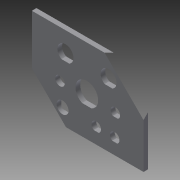
# Autodesk Inventor part: Yagi_Front_BackPlate
Saved by Autodesk Inventor 2014 (Build 180170000, 170)
## iProperties
Created: 2015-01-07
Part Number: Yagi_Front_BackPlate
Material: Generic
Document SubType Name: Modeling
Designer: Owner
Density: 1 g/cm^3
Appearance: Default
Author: Owner
Autodesk Inventor part; units mm, degrees
ref_plane "YZ Plane" through (0, 0, 0) normal (1, 0, 0) x (0, 1, 0)
ref_plane "XZ Plane" through (0, 0, 0) normal (0, 1, 0) x (-1, 0, 0)
ref_plane "XY Plane" through (0, 0, 0) normal (0, 0, 1) x (1, 0, 0)
sketch "Sketch1" plane through (0, 0, 0) normal (0, 0, 1) x (1, 0, 0)
  line L0 (-24.8346, -36.7982) -> (51.3654, -36.7982)
  line L1 (51.3654, -36.7982) -> (51.3654, -93.9482)
  line L2 (51.3654, -93.9482) -> (-24.8346, -93.9482)
  line L3 (-24.8346, -93.9482) -> (-24.8346, -36.7982)
  point P0 (0, 0)
  dimension "d0" = 76.2
  dimension "d1" = 57.15
  constraints: 8 end point, 2 parallel, 1 horizontal, 1 perpendicular
  measures "d0" distance of L0.start L0.end
  measures "d1" distance of L0.end L1.end
extrude "Extrusion1" add sketch "Sketch1" along normal blind 3.175
sketch "Sketch2" plane through (0, 0, 0) normal (0, 0, -1) x (-1, 0, 0)
  line L0 (24.8346, -93.9482) -> (24.8346, -36.7982) projected
  line L1 (-51.3654, -93.9482) -> (24.8346, -93.9482) projected
  circle A0 centre (-27.529, -50.54) radius 9.0932 construction
  arc A1 (-24.7899, -55.2644) -> (-30.2681, -55.2644) centre (-27.529, -50.54) ccw
  line L2 (-30.2681, -55.2644) -> (-24.7899, -55.2644)
  circle A2 centre (-12.6895, -67.132) radius 10.3124 construction
  arc A3 (-9.447, -74.1678) -> (-15.9319, -74.1678) centre (-12.6895, -67.132) ccw
  line L3 (-15.9319, -74.1678) -> (-9.447, -74.1678)
  circle A4 centre (1.9171, -50.54) radius 9.0932 construction
  arc A5 (4.6562, -55.2644) -> (-0.822, -55.2644) centre (1.9171, -50.54) ccw
  line L4 (-0.822, -55.2644) -> (4.6562, -55.2644)
  circle A6 centre (3.8538, -83.4188) radius 4.1
  circle A7 centre (3.8538, -83.4188) radius 5.25 construction
  line L5 (24.8346, -54.8925) -> (24.8346, -40.8771)
  line L6 (24.8346, -36.7982) -> (-51.3654, -36.7982) projected
  arc A8 (-29.9902, -86.1688) -> (-33.4543, -86.1688) centre (-31.7222, -83.4188) ccw
  line L7 (-29.9902, -86.1688) -> (-33.4543, -86.1688)
  circle A9 centre (-31.7222, -83.4188) radius 5.5 construction
  arc A10 (-30.4636, -71.2982) -> (-33.9278, -71.2982) centre (-32.1957, -68.5482) ccw
  line L8 (-30.4636, -71.2982) -> (-33.9278, -71.2982)
  circle A11 centre (-32.1957, -68.5482) radius 5.5 construction
  arc A12 (3.8538, -65.7982) -> (7.3179, -65.7982) centre (5.5858, -68.5482) ccw
  line L9 (3.8538, -65.7982) -> (7.3179, -65.7982)
  circle A13 centre (5.5858, -68.5482) radius 5.5 construction
  arc A14 (-17.3964, -86.1688) -> (-20.8605, -86.1688) centre (-19.1284, -83.4188) ccw
  line L10 (-17.3964, -86.1688) -> (-20.8605, -86.1688)
  circle A15 centre (-19.1284, -83.4188) radius 5.5 construction
  line L11 (-51.3654, -36.7982) -> (-51.3654, -93.9482) projected
  line L12 (-45.0154, -36.7982) -> (-45.0154, -93.9482) construction
  line L13 (12.1346, -93.9482) -> (12.1346, -36.7982) construction
  line L14 (-51.3654, -90.7732) -> (24.8346, -90.7732) construction
  line L15 (-51.3654, -39.9732) -> (24.8346, -39.9732) construction
  point P0 (0, 0)
  dimension "d28" = 18.1864
  dimension "d29" = 10.922
  dimension "d30" = 4.7244
  dimension "d31" = 20.6248
  dimension "d32" = 15.494
  dimension "d33" = 7.0358
  dimension "d34" = 18.1864
  dimension "d35" = 10.922
  dimension "d36" = 4.7244
  dimension "d41" = 8.2
  dimension "d42" = 10.5
  dimension "d49" = 6.5
  dimension "d53" = 2.75
  dimension "d54" = 11
  dimension "d55" = 0
  dimension "d56" = 6.5
  dimension "d57" = 2.75
  dimension "d58" = 11
  dimension "d59" = 0
  dimension "d60" = 6.5
  dimension "d61" = 2.75
  dimension "d62" = 11
  dimension "d63" = 0
  dimension "d64" = 6.5
  dimension "d65" = 2.75
  dimension "d66" = 11
  dimension "d67" = 0
  dimension "d68" = 6.35
  dimension "d69" = 12.7
  dimension "d70" = 3.175
  dimension "d71" = 3.175
  dimension "d72" = 25.4
  dimension "d73" = 25.4
  dimension "d74" = 44.3303
  dimension "d75" = 24.8241
  dimension "d76" = 6.5488
  dimension "d77" = 8.2809
  dimension "d78" = 31.263
  dimension "d79" = 43.8569
  dimension "d80" = 10.2175
  dimension "d81" = 39.6636
  constraints: 24 end point, 16 centre point, 14 point on circle, 9 parallel, 9 point on line, 4 coincident, 2 perpendicular
  measures "d28" diameter of A0
  measures "d29" diameter of A1
  measures "d30" distance from line of L2 A1.centre
  measures "d31" diameter of A2
  measures "d32" diameter of A3
  measures "d33" distance from line of A3.centre L3
  measures "d34" diameter of A4
  measures "d35" diameter of A5
  measures "d36" distance from line of L4 A5.centre
  measures "d41" diameter of A6
  measures "d42" diameter of A7
  measures "d49" diameter of A8
  measures "d53" distance from line of L7 A8.centre
  measures "d54" diameter of A9
  measures "d55" distance of A9.centre A8.centre
  measures "d56" diameter of A10
  measures "d57" distance from line of L8 A10.centre
  measures "d58" diameter of A11
  measures "d59" distance of A11.centre A10.centre
  measures "d60" diameter of A12
  measures "d61" distance from line of L9 A12.centre
  measures "d62" diameter of A13
  measures "d63" distance of A13.centre A12.centre
  measures "d64" diameter of A14
  measures "d65" distance from line of L10 A14.centre
  measures "d66" diameter of A15
  measures "d67" distance of A15.centre A14.centre
  measures "d68" distance between parallel lines of L11 L12
  measures "d69" distance between parallel lines of L0 L13
  measures "d70" distance between parallel lines of L1 L14
  measures "d71" distance between parallel lines of L6 L15
  measures "d72" distance from line of L1 A13.centre
  measures "d73" distance from line of L1 A10.centre
  measures "d74" distance from line of L13 A11.centre
  measures "d75" distance from line of L13 A2.centre
  measures "d76" distance from line of L13 A12.centre
  measures "d77" distance from line of L13 A6.centre
  measures "d78" distance from line of L13 A15.centre
  measures "d79" distance from line of L13 A8.centre
  measures "d80" distance from line of A4.centre L13
  measures "d81" distance from line of L13 A0.centre
extrude "Extrusion2" cut sketch "Sketch2" against normal blind 6.35 contours L2 A1 | L3 A3 | L4 A5 | A6 | L7 A8 | L8 A10 | L9 A12 | L10 A14
body "Solid1"
